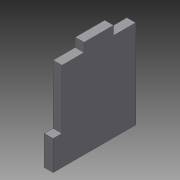
# Autodesk Inventor part: Motor side
Saved by Autodesk Inventor 2015 (Build 190159000, 159)
## iProperties
Created: 2014-07-26
Part Number: Motor side
Material: Generic
Document SubType Name: Modeling
Designer: karl
Density: 1 g/cm^3
Appearance: Default
Author: karl
Autodesk Inventor part; units mm, degrees
ref_plane "YZ Plane" through (0, 0, 0) normal (1, 0, 0) x (0, 1, 0)
ref_plane "XZ Plane" through (0, 0, 0) normal (0, 1, 0) x (-1, 0, 0)
ref_plane "XY Plane" through (0, 0, 0) normal (0, 0, 1) x (1, 0, 0)
sketch "Sketch1" plane through (0, 0, 0) normal (1, 0, 0) x (0, 1, 0)
  line L0 (-12.5, -15) -> (12.5, -15)
  line L1 (12.5, -15) -> (12.5, 15)
  line L2 (12.5, 15) -> (-12.5, 15)
  line L3 (-12.5, 15) -> (-12.5, -15)
  line L4 (-12.5, -15) -> (12.5, 15) construction
  line L5 (12.5, -15) -> (-12.5, 15) construction
  line L6 (5, 15) -> (-5, 15)
  line L7 (-5, 15) -> (-5, 18)
  line L8 (-5, 18) -> (5, 18)
  line L9 (5, 18) -> (5, 15)
  line L10 (-12.5, -15) -> (-15.5, -15)
  line L11 (-15.5, -15) -> (-15.5, -5)
  line L12 (-15.5, -5) -> (-12.5, -5)
  line L13 (-12.5, -5) -> (-12.5, -15)
  line L14 (12.5, -15) -> (15.5, -15)
  line L15 (15.5, -15) -> (15.5, -5)
  line L16 (15.5, -5) -> (12.5, -5)
  line L17 (12.5, -5) -> (12.5, -15)
  point P0 (0, 0)
  point P1 (0, 18)
  point P2 (0, 0)
  dimension "d0" = 25
  dimension "d1" = 10
  dimension "d2" = 3
  dimension "d3" = 3
  dimension "d4" = 10
  dimension "d5" = 20
  dimension "d8" = 3
  constraints: 36 end point, 8 parallel, 4 horizontal, 4 midpoint, 4 perpendicular, 1 collinear, 1 point on line, 1 vertical alignment
  measures "d0" distance of L2.end L1.end
  measures "d1" distance of L7.end L8.end
  measures "d2" distance of L6.end L7.end
  measures "d3" distance of L11.end L12.end
  measures "d4" distance of L10.end L11.end
  measures "d5" distance between parallel lines of L2 L12
  measures "d8" distance of L16.end L15.end
extrude "Extrusion1" add sketch "Sketch1" along normal blind 3
body "Solid1"
